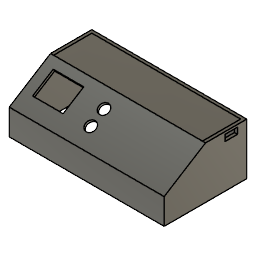
ars (Autodesk Fusion 360 archive; units mm, degrees)
design "utama"
Autodesk Fusion 360 part; units mm, degrees
sketch "Sketch3" plane through (0, 0, 0) normal (0, 0, 1) x (1, 0, 0)
  line L0 (75, 40) -> (-75, 40)
  line L1 (-75, 40) -> (-75, -40)
  line L2 (-75, -40) -> (75, -40)
  line L3 (75, -40) -> (75, 40)
  line L4 (75, 40) -> (-75, -40) construction
  line L5 (-75, 40) -> (75, -40) construction
  line L6 (-72, -37) -> (72, -37)
  line L7 (72, -37) -> (72, 37)
  line L8 (72, 37) -> (-72, 37)
  line L9 (-72, 37) -> (-72, -37)
  dimension "d8" = 150
  dimension "d9" = 80
  dimension "d10" = -3
  constraint horizontal L0
  constraint perpendicular L0 L1
  constraint parallel L0 L2
  constraint parallel L1 L3
  constraint coincident L4 origin
  constraint coincident L5 origin
  measures "d8" distance of L1.end L2.end
  measures "d9" distance of L0.end L1.end
extrude "Extrude2" add sketch "Sketch3" along normal blind 50
sketch "Sketch5" plane through (75, 0, 0) normal (1, 0, 0) x (0, 1, 0)
  line L0 (-40, 0) -> (40, 0)
  line L1 (40, 0) -> (40, 50)
  line L2 (40, 50) -> (-40, 50)
  line L3 (-40, 50) -> (-40, 0)
  line L4 (0, 50) -> (-40, 25)
  constraint midpoint L2 L4.start
  constraint midpoint L3 L4.end
extrude "Extrude3" cut sketch "Sketch5" against normal blind 150 contours L2 L3 L4
sketch "Sketch6" plane through (-72, 0, 0) normal (1, 0, 0) x (0, 1, 0)
  line L0 (-37, 26.875) -> (-37, 0)
  line L1 (-37, 0) -> (37, 0)
  line L2 (37, 0) -> (37, 50)
  line L3 (37, 50) -> (0, 50)
  line L4 (0, 50) -> (-37, 26.875)
  line L5 (0, 50) -> (0, 49.9999)
  line L6 (-37, 26.875) -> (-37, 23.875)
  line L7 (0, 50) -> (37, 50)
  line L8 (0, 49.9999) -> (37, 49.9999)
  line L9 (37, 49.9999) -> (37, 50)
  line L10 (0, 50) -> (-37, 26.875)
  line L11 (0, 50) -> (0, 47)
  line L12 (0, 47) -> (-37, 23.875)
  line L13 (-37, 26.875) -> (0, 50)
  line L14 (0, 50) -> (37, 50)
  line L15 (37, 50) -> (37, 47)
  line L16 (0, 47) -> (37, 47)
  dimension "d15" = 3
  dimension "d40" = 3
  dimension "d41" = 3
  constraint coincident L3.end L4.start
  constraint coincident L0.start L4.end
  constraint perpendicular L3 L5
  constraint parallel L0 L6
  constraint coincident L2.end L3.start
  constraint coincident L2 L8.end
  constraint perpendicular L2 L8
  constraint perpendicular L3 L11
  constraint coincident L2 L15.end
  measures "d15" distance of L0.start L6.end
  measures "d40" distance of L3.end L11.end
  measures "d41" distance of L2.end L15.end
extrude "Extrude4" add sketch "Sketch6" along normal blind 145 contours L0 L4 L6 L10 L11 L12 L13 | L2 L3 L7 L8 L11 L14 L15 L16
sketch "Sketch7" plane through (0, -22.4719, 35.9551) normal (0, -0.529999, 0.847998) x (1, 0, 0)
  line L0 (75, 26.4999) -> (72, 26.4999)
  line L1 (-75, -20.67) -> (75, -20.67)
  line L2 (75, -20.67) -> (75, 26.4999)
  line L3 (-65, 17.83) -> (-35.5, 17.83)
  line L4 (-35.5, 17.83) -> (-35.5, -5.67)
  line L5 (-35.5, -5.67) -> (-65, -5.67)
  line L6 (-65, -5.67) -> (-65, 17.83)
  line L7 (72, 26.4999) -> (-72, 26.4999)
  line L8 (-72, 26.4999) -> (-75, 26.4999)
  line L9 (-75, 26.4999) -> (-75, -20.67)
  dimension "d22" = 23.5
  dimension "d23" = 29.5
  dimension "d42" = 10
  dimension "d43" = 15
  constraint horizontal L3
  constraint vertical L4
  constraint horizontal L5
  constraint vertical L6
  measures "d22" distance of L3.end L4.end
  measures "d23" distance of L3.start L3.end
  measures "d42" distance of L6 L9
  measures "d43" distance of L1 L5
extrude "Extrude6" cut sketch "Sketch7" against normal blind 15 contours L3 L4 L5 L6
sketch "Sketch9" plane through (0, 0, 50) normal (0, 0, 1) x (-1, 0, 0)
  line L0 (75, 0) -> (72, 0)
  line L1 (-75, 0) -> (-75, -40)
  line L2 (-75, -40) -> (75, -40)
  line L3 (75, -40) -> (75, 0)
  line L4 (72, 0) -> (72, -37)
  line L5 (72, -37) -> (-72, -37)
  line L6 (-72, -37) -> (-72, 0)
  line L7 (-72, 0) -> (-75, 0)
sketch "Sketch10" plane through (0, -22.4719, 35.9551) normal (0, -0.529999, 0.847998) x (1, 0, 0)
  line L0 (-35.5, 17.83) -> (-35.5, -5.67)
  line L1 (-35.5, -5.67) -> (-65, -5.67)
  line L2 (-65, -5.67) -> (-65, 17.83)
  line L3 (-65, 17.83) -> (-35.5, 17.83)
  line L4 (75, 26.4999) -> (72, 26.4999)
  circle A0 centre (-10.5, 11.4999) radius 5
  circle A1 centre (-10.5, -3.67) radius 5
  line L5 (72, 26.4999) -> (-72, 26.4999)
  line L6 (-72, 26.4999) -> (-75, 26.4999)
  line L7 (-75, 26.4999) -> (-75, -20.67)
  line L8 (-75, -20.67) -> (75, -20.67)
  line L9 (75, -20.67) -> (75, 26.4999)
  dimension "d25" = 10
  dimension "d44" = 25
  dimension "d45" = 25
  dimension "d46" = 17
  dimension "d47" = 15
  measures "d25" diameter of A0
  measures "d44" distance of L0 A0.centre
  measures "d45" distance of L0 A1.centre
  measures "d46" distance of A1.centre L8
  measures "d47" distance of A0.centre L5
extrude "Extrude7" cut sketch "Sketch10" against normal blind 5 contours A0 | A1
sketch "Sketch11" plane through (0, -22.4719, 35.9551) normal (0, -0.529999, 0.847998) x (1, 0, 0)
  circle A0 centre (-10.5, 11.4999) radius 5
  circle A1 centre (-10.5, -3.67) radius 5
  line L0 (-35.5, 17.83) -> (-35.5, -5.67)
  line L1 (-35.5, -5.67) -> (-65, -5.67)
  line L2 (-65, -5.67) -> (-65, 17.83)
  line L3 (-65, 17.83) -> (-35.5, 17.83)
  line L4 (75, 26.4999) -> (72, 26.4999)
  line L5 (72, 26.4999) -> (-72, 26.4999)
  line L6 (-72, 26.4999) -> (-75, 26.4999)
  line L7 (-75, 26.4999) -> (-75, -20.67)
  line L8 (-75, -20.67) -> (75, -20.67)
  line L9 (75, -20.67) -> (75, 26.4999)
sketch "Sketch12" plane through (75, 0, 0) normal (1, 0, 0) x (0, 1, 0)
  line L0 (0, 50) -> (-40, 25)
  line L1 (-40, 25) -> (-40, 0)
  line L2 (-40, 0) -> (40, 0)
  line L3 (40, 0) -> (40, 50)
  line L4 (40, 50) -> (0, 50)
  line L5 (19, 47.7047) -> (31, 47.7047)
  line L6 (31, 47.7047) -> (31, 41.7047)
  line L7 (31, 41.7047) -> (19, 41.7047)
  line L8 (19, 41.7047) -> (19, 47.7047)
  point P0 (0, 50)
  point P1 (40, 50)
  dimension "d32" = 40
  dimension "d33" = 12
  dimension "d34" = 6
  dimension "d35" = 9
  constraint horizontal L5
  constraint vertical L6
  constraint horizontal L7
  constraint vertical L8
  measures "d32" distance of P0 P1
  measures "d33" distance of L5.start L5.end
  measures "d34" distance of L5.start L7.end
  measures "d35" distance of L3 L5.end
extrude "Extrude8" cut sketch "Sketch12" against normal blind 5 contours L5 L6 L7 L8
sketch "Sketch13" plane through (75, 0, 0) normal (1, 0, 0) x (0, 1, 0)
  line L0 (31, 47.7047) -> (31, 41.7047)
  line L1 (31, 41.7047) -> (19, 41.7047)
  line L2 (19, 41.7047) -> (19, 47.7047)
  line L3 (19, 47.7047) -> (31, 47.7047)
  line L4 (0, 50) -> (-40, 25)
  line L5 (-40, 25) -> (-40, 0)
  line L6 (-40, 0) -> (40, 0)
  line L7 (40, 0) -> (40, 50)
  line L8 (40, 50) -> (0, 50)
sketch "Sketch14" plane through (0, -22.4719, 35.9551) normal (0, -0.529999, 0.847998) x (1, 0, 0)
  line L0 (9.0692, 33.0905) -> (68.0692, 33.0905)
  line L1 (68.0692, 33.0905) -> (68.0692, -5.9095)
  line L2 (68.0692, -5.9095) -> (9.0692, -5.9095)
  line L3 (9.0692, -5.9095) -> (9.0692, 33.0905)
  dimension "d38" = 59
  dimension "d39" = 39
  constraint horizontal L0
  constraint vertical L1
  constraint horizontal L2
  constraint vertical L3
  measures "d38" distance of L0.start L0.end
  measures "d39" distance of L0.start L2.end
